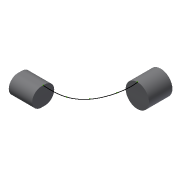
# Autodesk Inventor part: loft
Saved by Autodesk Inventor 2022 Beta2 (Build 260130000, 130) ContinuousBuild 0
## iProperties
Shininess: 64.0
Length Units: 11269
Angle Units: 11279
Time Units: 11290
Mass Units: 11283
Length Display Precision: 3
Angle Display Precision: 2
Compacted: True
Part Number: loft
Document SubType Name: Modeling
Created: 2002-11-25
Designer: Administrator
Density: 1 g/cm^3
Material: Generic
Appearance: Light Gray
Density: 0.0
Volumn: 0.0
Area: 0.0
PropertySet Name: Model Information
Control State: 0
Master: False
Checked Out: False
Author: Administrator
Autodesk Inventor part; units mm, degrees
ref_plane "YZ Plane" through (0, 0, 0) normal (1, 0, 0) x (0, 1, 0)
sketch "Sketch1" plane through (0, 0, 0) normal (0, 0, 1) x (1, 0, 0)
  circle A0 centre (0, 0) radius 12.7
  dimension "d0" = 25.4
  constraints: 1 centre point
  measures "d0" diameter of A0
extrude "Extrusion1" add sketch "Sketch1" along normal blind 25.4
sketch "Sketch2" plane through (0, 0, 25.4) normal (0, 0, 1) x (1, 0, 0)
  circle A0 centre (0, 0) radius 12.7 projected
  line L0 (0, 12.7) -> (0, -12.7)
  constraints: 2 end point, 2 point on circle, 1 vertical, 1 vertical alignment
ref_plane "Work Plane1" through (0, 12.7, 25.4) normal (-1, 0, 0) x (0, -1, 0)
ref_plane "Work Plane2" through (-50.8, 12.7, 25.4) normal (-1, 0, 0) x (0, -1, 0)
sketch "Sketch3" plane through (-50.8, 12.7, 25.4) normal (-1, 0, 0) x (0, -1, 0)
  line L0 (0, -25.4) -> (0, 0) projected
  line L1 (0, 0) -> (25.4, 0) projected
  line L2 (2.7, 53.6) -> (2.7, 49.6)
  arc A0 (2.7, 49.6) -> (22.7, 49.6) centre (12.7, 49.6) ccw
  line L3 (22.7, 49.6) -> (22.7, 53.6)
  arc A1 (22.7, 53.6) -> (2.7, 53.6) centre (12.7, 53.6) ccw
  line L4 (12.7, -43.9769) -> (12.7, 86.0616) projected
  line L5 (-27.2073, -25.4) -> (39.5727, -25.4) projected
  dimension "d88" = 10
  dimension "d89" = 4
  dimension "d90" = 75
  constraints: 4 end point, 4 point on circle, 3 tangent, 2 centre point, 1 equal radius, 1 parallel, 1 perpendicular, 1 point on line
  measures "d88" radius of A0
  measures "d89" distance of A1.centre A0.centre
  measures "d90" distance from line of A0.centre L5
extrude "Extrusion2" add sketch "Sketch3" along normal blind 25.4 contours A0 L2 A1 L4 | L4 A1 L3 A0
shell "Shell1" thickness 1 removed faces 2 at (-3.6254, -0.9542, 0) at (-76.2, -0.4018, 71.691)
sketch3d "3D Sketch4"
body "Solid1"
